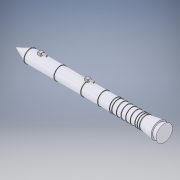
# Autodesk Inventor part: bost
Saved by Autodesk Inventor 2018 (Build 220112000, 112)
## iProperties
Created: 2017-09-24
Part Number: bost
Material: Generic
Document SubType Name: Modeling
Designer: akshay.biju
Density: 1 g/cm^3
Appearance: Default
Author: akshay.biju
Autodesk Inventor part; units mm, degrees
ref_plane "YZ Plane" through (0, 0, 0) normal (1, 0, 0) x (0, 1, 0)
ref_plane "XY Plane" through (0, 0, 0) normal (0, 0, 1) x (1, 0, 0)
sketch "Sketch1" plane through (0, 0, 0) normal (0, 1, 0) x (-1, 0, 0)
  line L0 (0, 0) -> (450, 0)
  line L1 (0, 0) -> (0, 25)
  line L2 (15, 0) -> (15, 25)
  line L3 (15, 20) -> (0, 25)
  line L4 (55, 0) -> (55, 20)
  line L5 (55, 20) -> (56, 20)
  line L6 (55, 20) -> (56, 20) construction
  line L7 (56, 20) -> (56, 0)
  line L8 (55, 18.75) -> (15, 25)
  line L9 (56, 0) -> (56, -0.5979)
  line L10 (56, 0) -> (62, 0)
  line L11 (62, 0) -> (62, 20)
  line L12 (62, 18.75) -> (56, 18.75)
  line L13 (62, 20) -> (63, 20)
  line L14 (63, 20) -> (63, 0)
  line L15 (63, 0) -> (69, 0)
  line L16 (69, 0) -> (69, 20)
  line L17 (69, 20) -> (70, 20)
  line L18 (70, 20) -> (70, 0)
  line L19 (69, 18.75) -> (63, 18.75)
  line L20 (70, 18.75) -> (83, 18.75)
  line L21 (83, 18.75) -> (83, 0)
  line L22 (83, 0) -> (84, 0)
  line L23 (84, 0) -> (84, 20)
  line L24 (84, 20) -> (83, 20)
  line L25 (83, 20) -> (83, 18.75)
  line L26 (84, 18.75) -> (97, 18.75)
  line L27 (97, 18.75) -> (97, 0)
  line L28 (97, 0) -> (98, 0)
  line L29 (98, 0) -> (98, 20)
  line L30 (98, 20) -> (97, 20)
  line L31 (97, 20) -> (97, 18.75)
  line L32 (98, 18.75) -> (111, 18.75)
  line L33 (111, 18.75) -> (111, 0)
  line L34 (111, 0) -> (112, 0)
  line L35 (112, 0) -> (112, 20)
  line L36 (112, 20) -> (111, 20)
  line L37 (111, 20) -> (111, 18.75)
  line L38 (126, 0) -> (139, 0)
  line L39 (112, 18.75) -> (125, 18.75)
  line L40 (125, 18.75) -> (125, 0)
  line L41 (125, 0) -> (126, 0)
  line L42 (126, 0) -> (126, 20)
  line L43 (126, 20) -> (125, 20)
  line L44 (125, 20) -> (125, 18.75)
  line L45 (126, 18.75) -> (139, 18.75)
  line L46 (139, 18.75) -> (139, 0)
  line L47 (139, 0) -> (140, 0)
  line L48 (140, 0) -> (140, 20)
  line L49 (140, 20) -> (139, 20)
  line L50 (139, 20) -> (139, 18.75)
  line L51 (140, 18.75) -> (146, 18.75)
  line L52 (146, 18.75) -> (146, 0)
  line L53 (146, 0) -> (147, 0)
  line L54 (147, 0) -> (147, 20)
  line L55 (147, 20) -> (146, 20)
  line L56 (146, 20) -> (146, 18.75)
  line L57 (147, 18.75) -> (182, 18.75)
  line L58 (182, 18.75) -> (182, 0)
  line L59 (182, 0) -> (183, 0)
  line L60 (183, 0) -> (183, 20)
  line L61 (183, 20) -> (182, 20)
  line L62 (182, 20) -> (182, 18.75)
  line L63 (183, 18.75) -> (233, 18.75)
  line L64 (233, 18.75) -> (233, 0)
  line L65 (233, 0) -> (234, 0)
  line L66 (234, 0) -> (234, 20)
  line L67 (234, 20) -> (233, 20)
  line L68 (233, 20) -> (233, 18.75)
  line L69 (234, 0) -> (314, 0)
  line L70 (314, 0) -> (314, 20)
  line L71 (314, 18.75) -> (234, 18.75)
  line L72 (314, 20) -> (315, 20)
  line L73 (315, 20) -> (315, 0)
  line L74 (315, 18.75) -> (405, 18.75)
  line L75 (315, 18.75) -> (314.5, 18.75)
  line L76 (405, 18.75) -> (405, 0)
  line L77 (405, 18.75) -> (405, 20)
  line L78 (405, 20) -> (406, 20)
  line L79 (406, 20) -> (406, 0)
  line L80 (450, 0) -> (406, 18.75)
  constraints: 160 end point, 32 perpendicular, 26 point on line, 13 horizontal, 7 vertical, 2 collinear, 1 parallel, 29 other
revolve "Revolution1" add sketch "Sketch1" angle 360 about axis through (0, 0, 0) along (-1, 0, 0)
ref_plane "Work Plane1" through (-274, 18.75, 0) normal (0, 1, 0) x (-1, 0, 0)
sketch "Sketch3" plane through (-274, 18.75, 0) normal (0, 1, 0) x (-1, 0, 0)
  line L0 (132, 18.75) -> (176, 0) projected
  line L1 (176, 0) -> (95, 0)
  line L2 (105, -5) -> (105, 5)
  line L3 (105, 5) -> (95, 5)
  line L4 (95, 5) -> (95, -5)
  line L5 (95, -5) -> (105, -5)
  point P0 (-274, 0)
  point P1 (100, 0)
  constraints: 10 end point, 2 parallel, 2 perpendicular, 1 horizontal, 1 point on line
extrude "Extrusion1" add sketch "Sketch3" along normal blind 7.5
sketch "Sketch4" plane through (-369, 18.75, 5) normal (1, 0, 0) x (0, 0, -1)
  circle A0 centre (5, 5) radius 2.5
  point P0 (5, -18.75)
  constraints: 1 centre point
extrude "Extrusion2" add sketch "Sketch4" along normal blind 13
sketch "Sketch5" plane through (-274, 18.75, 0) normal (0, 1, 0) x (-1, 0, 0)
  line L0 (105, -5) -> (105, 5) projected
  line L1 (105, 0) -> (-35, 0)
  line L2 (95, 0) -> (105, 0) projected
  line L3 (-35, 0) -> (-45, 0)
  line L4 (-45, -7.3429) -> (-35, -7.3429)
  line L5 (-35, -7.3429) -> (-35, 2.6571)
  line L6 (-35, 2.6571) -> (-45, 2.6571)
  line L7 (-45, 2.6571) -> (-45, -7.3429)
  line L8 (-45, -7.3429) -> (-35, 2.6571) construction
  line L9 (-35, -7.3429) -> (-45, 2.6571) construction
  line L10 (-41, -20) -> (-41, 20) projected
  point P0 (-274, 0)
  point P1 (-40, -2.3429)
  dimension "d77" = 140
  dimension "d78" = 10
  dimension "d79" = 10
  constraints: 16 end point, 3 midpoint, 2 parallel, 2 perpendicular, 1 collinear, 1 horizontal
  measures "d77" distance of L1.start L1.end
  measures "d78" distance of L1.end L3.end
  measures "d79" distance of L5.end L4.end
extrude "Extrusion3" add sketch "Sketch5" along normal blind 7.5
sketch "Sketch6" plane through (-229, 18.75, 0) normal (1, 0, 0) x (0, 0, -1)
  circle A0 centre (2.5, 5) radius 2.5
  point P0 (0, -18.75)
  dimension "d82" = 5
  constraints: 1 centre point
  measures "d82" diameter of A0
extrude "Extrusion4" add sketch "Sketch6" along normal blind 13
body "Solid1"
